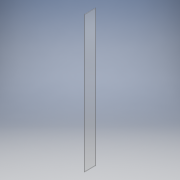
# Autodesk Inventor part: Ground_Antenna230mm_Support
Saved by Autodesk Inventor 2018 (Build 220112000, 112)
## iProperties
Created: 2018-09-26
Part Number: Ground_Antenna230mm_Support
Material: Polycarbonate, Clear
Document SubType Name: Modeling
Designer: Bradley
Mass: 1764.56 g
Surface Area: 6314.01 cm^2
Volume: 1470.47 cm^3
Density: 1.2 g/cm^3
Appearance: Polycarbonate - Clear
Author: Bradley
Autodesk Inventor part; units mm, degrees
ref_plane "YZ Plane" through (0, 0, 0) normal (1, 0, 0) x (0, 1, 0)
ref_plane "XZ Plane" through (0, 0, 0) normal (0, 1, 0) x (-1, 0, 0)
ref_plane "XY Plane" through (0, 0, 0) normal (0, 0, 1) x (1, 0, 0)
sketch "Sketch1" plane through (0, 0, 0) normal (1, 0, 0) x (0, 1, 0)
  line L0 (-49.4, -600) -> (49.4, -600)
  line L1 (49.4, -600) -> (49.4, 600)
  line L2 (49.4, 600) -> (-49.4, 600)
  line L3 (-49.4, 600) -> (-49.4, -600)
  line L4 (-49.4, -600) -> (49.4, 600) construction
  line L5 (49.4, -600) -> (-49.4, 600) construction
  line L6 (-42.4, 600) -> (-42.4, -600) construction
  line L7 (42.4, -600) -> (42.4, 600) construction
  line L8 (-42.4, 600) -> (42.4, 600) construction
  point P0 (0, 0)
  point P1 (0, 600)
  dimension "d0" = 84.8
  dimension "d1" = 7
  dimension "d2" = 1200
  constraints: 18 end point, 4 midpoint, 4 point on line, 3 perpendicular, 2 parallel, 1 collinear, 1 horizontal
  measures "d0" distance between parallel lines of L7 L6
  measures "d1" distance between parallel lines of L3 L6
  measures "d2" distance of L2.end L0.start
extrude "Extrusion1" add sketch "Sketch1" along normal mid plane 4.7625
body "Solid1"
